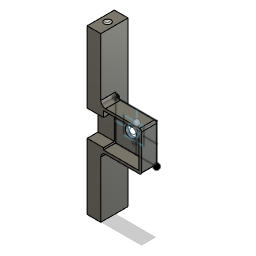
Держатель под камеру v7 (Autodesk Fusion 360 design; units mm, degrees)
Autodesk Fusion 360 part; units mm, degrees
sketch "Sketch1" plane through (0, 0, 0) normal (1, 0, 0) x (0, 1, 0)
  line L0 (0, 0) -> (-230, 0)
  line L1 (-230, 0) -> (-230, 150)
  line L2 (-230, 150) -> (0, 150)
  line L3 (0, 150) -> (0, 0)
  line L4 (-230, 0) -> (-220, 0)
  line L5 (-220, 0) -> (-220, 150)
  line L6 (-220, 150) -> (-230, 150)
  line L7 (-230, 150) -> (-230, 0)
  dimension "d1" = 230
  dimension "d2" = 150
  dimension "d3" = 10
  dimension "d4" = 150
  constraint horizontal L0
  constraint vertical L1
  constraint horizontal L2
  constraint vertical L3
  constraint coincident L0.start L3.end
  constraint horizontal L4
  constraint vertical L5
  constraint horizontal L6
  constraint vertical L7
  measures "d1" distance of L0.start L0.end
  measures "d2" distance of L0.start L2.end
  measures "d3" distance of L0.end L4.end
  measures "d4" distance of L0.end L1.end
extrude "Extrude1" add sketch "Sketch1" against normal blind 10
extrude "Extrude2" add 1 faces at (-6.6667, -230, 50) along direction (0, -1, 0) blind 20
extrude "Extrude3" add 1 faces at (-6.6667, 0, 100) along direction (0, 1, 0) blind 20
sketch "Sketch2" plane through (0, 0, 0) normal (1, 0, 0) x (0, 1, 0)
  line L0 (20, 150) -> (-250, 150)
  line L1 (-250, 150) -> (-250, 0)
  line L2 (-250, 0) -> (20, 0)
  line L3 (20, 0) -> (20, 150)
  line L4 (-250, 0) -> (-240, 0)
  line L5 (-240, 0) -> (-240, 15)
  line L6 (-240, 15) -> (-250, 15)
  line L7 (-250, 15) -> (-250, 0)
  line L8 (0, 0) -> (-10, 0)
  line L9 (-10, 0) -> (-10, 15)
  line L10 (-10, 15) -> (0, 15)
  line L11 (0, 15) -> (0, 0)
  dimension "d11" = 10
  dimension "d12" = 15
  dimension "d13" = 10
  dimension "d14" = 15
  dimension "d46" = 230
  constraint horizontal L4
  constraint vertical L5
  constraint horizontal L6
  constraint vertical L7
  constraint coincident L2 L1.end
  constraint horizontal L8
  constraint vertical L9
  constraint horizontal L10
  constraint vertical L11
  constraint coincident L8.start L11.end
  measures "d11" distance of L1.end L4.end
  measures "d12" distance of L1.end L6.end
  measures "d13" distance of L8.start L8.end
  measures "d14" distance of L8.start L10.end
  measures "d46" distance of L5 L9
extrude "Extrude12" add 1 faces at (-6.6667, -250, 50) along direction (0, -1, 0) blind 20
extrude "Extrude4" cut sketch "Sketch2" against normal blind 140 contours L1 L2 L4 L5 L6 L7 | L2 L8 L9 L10 L11
fillet "Fillet2" radius 20 1 edges at (-5, 20, 150)
sketch "Sketch3" plane through (0, 0, 0) normal (1, 0, 0) x (0, 1, 0)
  arc A0 (20, 130) -> (0, 150) centre (0, 130) ccw
  line L0 (0, 150) -> (-270, 150)
  line L1 (-250, 15) -> (-240, 15)
  line L2 (-240, 15) -> (-240, 0)
  line L3 (-270, 0) -> (-250, 0)
  line L4 (-10, 0) -> (-10, 15)
  line L5 (-10, 15) -> (0, 15)
  line L6 (0, 15) -> (0, 0)
  line L7 (0, 0) -> (20, 0)
  line L8 (20, 0) -> (20, 130)
  line L9 (-200, 0) -> (-30, 0)
  line L10 (-30, 0) -> (-30, 130)
  line L11 (-30, 130) -> (-200, 130)
  line L12 (-200, 130) -> (-200, 0)
  line L13 (-270, 150) -> (-270, 0)
  line L14 (-250, 0) -> (-250, 15)
  line L15 (-240, 0) -> (-10, 0)
  constraint horizontal L9
  constraint vertical L10
  constraint horizontal L11
  constraint vertical L12
  constraint coincident L3 L9.start
extrude "Extrude5" cut sketch "Sketch3" against normal blind 100 contours L9 L10 L11 L12 L15
sketch "Sketch4" plane through (0, 0, 150) normal (0, 0, 1) x (-1, 0, 0)
  line L0 (0, 0) -> (10, 0)
  line L1 (10, 0) -> (10, 270)
  line L2 (0, 270) -> (0, 0)
  line L3 (0, 140) -> (-30, 140)
  line L4 (-30, 140) -> (-30, 111)
  line L5 (-30, 111) -> (0, 111)
  line L6 (0, 111) -> (0, 140)
  line L7 (0, 140) -> (-30, 111)
  line L8 (-30, 140) -> (0, 111)
  line L9 (-2, 138) -> (-28, 138)
  line L10 (-28, 138) -> (-28, 113)
  line L11 (-28, 113) -> (-2, 113)
  line L12 (-2, 113) -> (-2, 138)
  line L13 (-2, 138) -> (-28, 113) construction
  line L14 (-28, 138) -> (-2, 113) construction
  line L15 (10, 270) -> (0, 270)
  point P0 (-15, 125.5)
  dimension "d23" = 30
  dimension "d24" = 29
  dimension "d25" = 26
  dimension "d26" = 25
  constraint horizontal L3
  constraint vertical L4
  constraint horizontal L5
  constraint vertical L6
  constraint coincident L2 L3.start
  constraint horizontal L9
  constraint perpendicular L9 L10
  constraint parallel L9 L11
  constraint parallel L10 L12
  constraint coincident L13 P0
  constraint coincident L14 P0
  constraint midpoint L8 P0
  measures "d23" distance of L3.start L3.end
  measures "d24" distance of L3.start L5.end
  measures "d25" distance of L10.end L11.end
  measures "d26" distance of L9.end L10.end
extrude "Extrude6" add sketch "Sketch4" against normal blind 10 contours L2 L6 L7 L8 L9 L11 L12 | L5 L7 L8 L11 | L3 L7 L8 L9 | L4 L7 L8 L9 L10 L11 | L7 L8 L11 | L7 L8 L9 L11 L12 | L7 L8 L9 | L7 L8 L9 L10 L11
extrude "Extrude7" cut sketch "Sketch4" against normal blind 8 contours L7 L8 L11 | L7 L8 L9 L11 L12 | L7 L8 L9 | L7 L8 L9 L10 L11
extrude "Extrude9" add 1 faces at (20, -120.6667, 140) along direction (0, 0, -1) blind 1
sketch "Sketch5" plane through (0, 0, 139) normal (0, 0, -1) x (1, 0, 0)
  line L0 (0, 140) -> (0, 111)
  line L1 (0, 111) -> (30, 111)
  line L2 (30, 111) -> (30, 140)
  line L3 (30, 140) -> (0, 140)
  circle A0 centre (13.026, 125.5717) radius 4
  line L4 (0, 111) -> (30, 111)
  line L5 (30, 111) -> (30, 140)
  line L6 (30, 140) -> (0, 140)
  line L7 (0, 140) -> (0, 111)
  line L8 (0, 126.0602) -> (5.9, 126.0602)
  line L9 (15.4722, 111) -> (15.4722, 119.2)
  line L10 (30, 125.5) -> (20.7, 125.5)
  line L11 (15, 140) -> (15, 131.8)
  line L12 (5.9, 119.2) -> (20.7, 119.2)
  line L13 (20.7, 119.2) -> (20.7, 131.8)
  line L14 (20.7, 131.8) -> (5.9, 131.8)
  line L15 (5.9, 131.8) -> (5.9, 119.2)
  dimension "d35" = 8
  dimension "d84" = 5.9
  dimension "d85" = 8.2
  dimension "d86" = 9.3
  dimension "d87" = 8.2
  constraint horizontal L4
  constraint vertical L5
  constraint horizontal L6
  constraint vertical L7
  constraint coincident L2.end L3.start
  constraint coincident L0.end L1.start
  constraint coincident L7 L8.start
  constraint perpendicular L7 L8
  constraint coincident L4 L9.start
  constraint perpendicular L4 L9
  constraint midpoint L5 L10.start
  constraint perpendicular L5 L10
  constraint midpoint L6 L11.start
  constraint perpendicular L6 L11
  constraint horizontal L12
  constraint vertical L13
  constraint horizontal L14
  constraint vertical L15
  constraint coincident L8.end L15
  constraint coincident L10.end L13
  measures "d35" diameter of A0
  measures "d84" distance of L8.start L8.end
  measures "d85" distance of L9.start L9.end
  measures "d86" distance of L10.start L10.end
  measures "d87" distance of L11.start L11.end
extrude "Extrude10" cut sketch "Sketch5" against normal blind 30 contours A0
fillet "Fillet3" radius 1.5 2 edges at (30, -111, 144.5) (30, -140, 144.5)
fillet "Fillet4" radius 3.5 1 edges at (0, -111, 144.5)
fillet "Fillet5" radius 3.5 1 edges at (0, -140, 144.5)
extrude "Extrude8" cut 1 faces at (24.342, -125.5239, 142) along direction (0, 0, -1) blind 1
fillet "Fillet7" radius 20 1 edges at (-5, -270, 150)
extrude "Extrude13" cut 1 faces at (-6.6667, -200, 86.6667) along direction (0, -1, 0) blind 20
fillet "Fillet8" radius 10 2 edges at (-5, -220, 130) (-5, -30, 130)
sketch "Sketch6" plane through (0, 0, 0) normal (1, 0, 0) x (0, 1, 0)
  line L0 (-210, 130) -> (-40, 130)
  arc A0 (-30, 120) -> (-40, 130) centre (-40, 120) ccw
  line L1 (-30, 120) -> (-30, 0)
  line L2 (-30, 0) -> (-10, 0)
  line L3 (-10, 0) -> (-10, 15)
  line L4 (-10, 15) -> (0, 15)
  line L5 (0, 15) -> (0, 0)
  line L6 (0, 0) -> (20, 0)
  line L7 (20, 0) -> (20, 130)
  arc A1 (20, 130) -> (0, 150) centre (0, 130) ccw
  line L8 (0, 150) -> (-107.5, 150)
  line L9 (-107.5, 150) -> (-107.5, 139)
  line L10 (-107.5, 139) -> (-143.5, 139)
  line L11 (-143.5, 139) -> (-143.5, 150)
  line L12 (-143.5, 150) -> (-250, 150)
  arc A2 (-250, 150) -> (-270, 130) centre (-250, 130) ccw
  line L13 (-270, 130) -> (-270, 0)
  line L14 (-270, 0) -> (-250, 0)
  line L15 (-250, 0) -> (-250, 15)
  line L16 (-250, 15) -> (-240, 15)
  line L17 (-240, 15) -> (-240, 0)
  line L18 (-240, 0) -> (-220, 0)
  line L19 (-220, 0) -> (-220, 120)
  arc A3 (-210, 130) -> (-220, 120) centre (-210, 120) ccw
  line L20 (-270, 0) -> (-198, 0)
  line L21 (-198, 0) -> (-198, 167.8427)
  line L22 (-198, 167.8427) -> (-270, 167.8427)
  line L23 (-270, 167.8427) -> (-270, 0)
  line L24 (20, 0) -> (-52, 0)
  line L25 (-52, 0) -> (-52, 156.7227)
  line L26 (-52, 156.7227) -> (20, 156.7227)
  line L27 (20, 156.7227) -> (20, 0)
  dimension "d57" = 72
  constraint horizontal L20
  constraint vertical L21
  constraint horizontal L22
  constraint vertical L23
  constraint coincident L13.end L14.start
  constraint horizontal L24
  constraint vertical L25
  constraint horizontal L26
  constraint vertical L27
  constraint coincident L6.end L7.start
  measures "d57" distance of L6.end L24.end
extrude "Extrude14" cut sketch "Sketch6" against normal blind 180 contours L0 L12 A2 L13 L14 L15 L16 L17 L18 L19 A3 L20 L21 L23 | L0 L19 A3 L20 L21 | L0 A0 L1 L2 L3 L4 L5 L6 L7 A1 L8 L24 L25 L27 | L0 A0 L1 L24 L25 | L12 A2 L21 L22 L23 | A1 L8 L25 L26 L27
sketch "Sketch7" plane through (0, 0, 0) normal (1, 0, 0) x (0, 1, 0)
  line L0 (-198, 150) -> (-198, 130)
  line L1 (-198, 130) -> (-52, 130)
  line L2 (-52, 130) -> (-52, 150)
  line L3 (-52, 150) -> (-107.5, 150)
  line L4 (-107.5, 150) -> (-107.5, 139)
  line L5 (-107.5, 139) -> (-143.5, 139)
  line L6 (-143.5, 139) -> (-143.5, 150)
  line L7 (-143.5, 150) -> (-198, 150)
  line L8 (-198, 150) -> (-250, 150)
  line L9 (-52, 150) -> (0, 150)
  line L10 (-250, 150) -> (-250, 130)
  line L11 (-250, 130) -> (-198, 130)
  line L12 (0, 150) -> (0, 130)
  line L13 (0, 130) -> (-52, 130)
  dimension "d60" = 52
  dimension "d61" = 52
  constraint coincident L0.start L7.end
  constraint perpendicular L2 L8
  constraint coincident L2.end L3.start
  constraint perpendicular L2 L9
  constraint perpendicular L8 L10
  constraint coincident L0.end L1.start
  constraint perpendicular L0 L11
  constraint perpendicular L1 L12
  constraint coincident L1.end L2.start
  constraint perpendicular L2 L13
  measures "d60" distance of L0.start L8.end
  measures "d61" distance of L2.end L9.end
extrude "Extrude15" add sketch "Sketch7" against normal blind 10 contours L0 L8 L10 L11 | L2 L9 L12 L13
sketch "Sketch8" plane through (0, -250, 0) normal (0, -1, 0) x (1, 0, 0)
  line L0 (0, 130) -> (0, 150)
  line L1 (0, 150) -> (-10, 150)
  line L2 (-10, 150) -> (-10, 130)
  line L3 (-10, 130) -> (0, 130)
  circle A0 centre (-5, 140) radius 3.5
  dimension "d64" = 7
  measures "d64" diameter of A0
extrude "Extrude16" cut sketch "Sketch8" against normal blind 20 contours A0
sketch "Sketch9" plane through (0, 0, 0) normal (0, 1, 0) x (-1, 0, 0)
  line L0 (0, 150) -> (0, 130)
  line L1 (0, 130) -> (10, 130)
  line L2 (10, 130) -> (10, 150)
  line L3 (10, 150) -> (0, 150)
  circle A0 centre (5, 140) radius 3.5
  dimension "d67" = 7
  measures "d67" diameter of A0
extrude "Extrude17" cut sketch "Sketch9" against normal blind 20 contours A0
thread "Thread1" "ISO Metric profile 7.0 M7x1 6H" major diameter 7.1472 minor diameter 6.0355 pitch 1 angle 60 resizes the face on face at (-1.7748, -13.3333, 138.6405)
thread "Thread2" "ISO Metric profile 7.0 M7x1 6H" major diameter 7.1472 minor diameter 6.0355 pitch 1 angle 60 resizes the face on face at (-8.2889, -236.6667, 138.8029)
extrude "Extrude18" cut 1 faces at (-4.9248, -250, 147.6698) along direction (0, 1, 0) blind 15
extrude "Extrude19" cut 1 faces at (-4.9248, 0, 147.6698) along direction (0, -1, 0) blind 15
extrude "Extrude20" cut 1 faces at (-4.9248, -235, 147.6698) along direction (0, 1, 0) blind 50
extrude "Extrude21" cut 1 faces at (-5.503, -230, 137.9955) along direction (0, 1, 0) blind 59
extrude "Extrude22" cut 1 faces at (-4.9248, -15, 147.6698) along direction (0, -1, 0) blind 50
extrude "Extrude23" cut 1 faces at (-4.497, -20, 137.9955) along direction (0, -1, 0) blind 57
extrude "Extrude24" add 1 faces at (-5.503, -171, 137.9955) along direction (0, -1, 0) blind 2
thread "Thread3" "ISO Metric profile 6.0 M6x1 6H" major diameter 6.147 minor diameter 5.035 pitch 1 angle 60 resizes the face on face at (-7.3117, -177, 138.0602)
thread "Thread4" "ISO Metric profile 6.0 M6x1 6H" major diameter 6.147 minor diameter 5.035 pitch 1 angle 60 resizes the face on face at (-2.5945, -73, 141.8221)
sketch "Sketch10" plane through (0, 0, 150) normal (0, 0, 1) x (-1, 0, 0)
  line L0 (-28, 138) -> (-2, 138)
  line L1 (-2, 138) -> (-2, 113)
  line L2 (-2, 113) -> (-28, 113)
  line L3 (-28, 113) -> (-28, 138)
  line L4 (0, 65) -> (10, 65)
  line L5 (10, 65) -> (10, 185)
  line L6 (10, 185) -> (0, 185)
  line L7 (0, 185) -> (0, 143.5)
  arc A0 (-3.5, 140) -> (0, 143.5) centre (-3.5, 143.5) ccw
  line L8 (-3.5, 140) -> (-28.5, 140)
  arc A1 (-28.5, 140) -> (-30, 138.5) centre (-28.5, 138.5) ccw
  line L9 (-30, 138.5) -> (-30, 112.5)
  arc A2 (-30, 112.5) -> (-28.5, 111) centre (-28.5, 112.5) ccw
  line L10 (-28.5, 111) -> (-3.5, 111)
  arc A3 (0, 107.5) -> (-3.5, 111) centre (-3.5, 107.5) ccw
  line L11 (0, 107.5) -> (0, 65)
  line L12 (-2, 117.3316) -> (10, 117.3316)
  line L13 (10, 117.3316) -> (10, 136.568)
  line L14 (10, 136.568) -> (-2, 136.568)
  line L15 (-2, 136.568) -> (-2, 117.3316)
  constraint horizontal L12
  constraint vertical L13
  constraint horizontal L14
  constraint vertical L15
  constraint coincident L5 L13.end
  constraint coincident L1 L12.start
extrude "Extrude25" cut sketch "Sketch10" against normal blind 8 contours L1 L5 L12 L13 L14 L15
